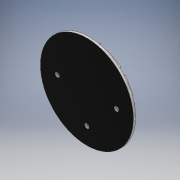
# Autodesk Inventor part: TSSP Receiver
Saved by Autodesk Inventor 2018 (Build 220112000, 112)
## iProperties
Created: 2018-09-04
Part Number: TSSP Receiver
Material: Generic
Document SubType Name: Modeling
Designer: matth
Density: 1 g/cm^3
Appearance: Default
Author: matth
Autodesk Inventor part; units mm, degrees
ref_plane "YZ Plane" through (0, 0, 0) normal (1, 0, 0) x (0, 1, 0)
ref_plane "XZ Plane" through (0, 0, 0) normal (0, 1, 0) x (-1, 0, 0)
ref_plane "XY Plane" through (0, 0, 0) normal (0, 0, 1) x (1, 0, 0)
sketch "Sketch1" plane through (0, 0, 0) normal (0, 1, 0) x (-1, 0, 0)
  line L0 (0, 0) -> (19.05, 0)
  line L1 (0, 0) -> (-19.05, 0)
  line L2 (0, 0) -> (0, -19.05)
  circle A0 centre (-19.05, 0) radius 1.5
  circle A1 centre (19.05, 0) radius 1.5
  circle A2 centre (0, -19.05) radius 1.5
  line L3 (0, -20.55) -> (0, -22.55)
  line L4 (0, -22.55) -> (5, -22.55)
  line L5 (5, -22.55) -> (5, -27.55)
  line L6 (5, -27.55) -> (-5, -27.55)
  line L7 (-5, -27.55) -> (-5, -22.55)
  line L8 (-5, -22.55) -> (0, -22.55)
  circle A3 centre (0, 0) radius 30
  dimension "d6" = 3
  dimension "d0" = 19.05
  dimension "d1" = 19.05
  dimension "d2" = 19.05
  dimension "d4" = 3
  dimension "d5" = 3
  dimension "d7" = 2
  dimension "d8" = 5
  dimension "d9" = 5
  dimension "d10" = 10
  dimension "d11" = 60
  constraints: 18 end point, 4 coincident, 3 centre point, 3 horizontal, 3 perpendicular, 2 vertical, 1 collinear, 1 point on line, 1 vertical alignment, 2 other
  measures "d0" distance of L0.start L0.end
  measures "d1" distance of L0.start L1.end
  measures "d2" distance of L0.start L2.end
  measures "d4" diameter of A0
  measures "d5" diameter of A1
  measures "d7" distance of L3.start L3.end
  measures "d8" distance of L3.end L4.end
  measures "d9" distance of L4.end L5.end
  measures "d10" distance of L5.end L6.end
  measures "d11" diameter of A3
extrude "Extrusion1" add sketch "Sketch1" along normal blind 1.5 contours L4 L5 L6 L7 L8 | A3
sketch "Sketch2" plane through (0, 1.5, 0) normal (0, 1, 0) x (1, 0, 0)
  line L0 (0, 0) -> (0, 22)
  line L1 (0, 22) -> (-5, 22)
  line L2 (-5, 22) -> (-5, 27)
  line L3 (-5, 27) -> (0, 27)
  line L4 (0, 27) -> (5, 27)
  line L5 (5, 27) -> (5, 22)
  line L6 (5, 22) -> (0, 22)
  line L7 (-11, 19.0526) -> (-15.3301, 16.5526)
  line L8 (-15.3301, 16.5526) -> (-17.8301, 20.8827)
  line L9 (-17.8301, 20.8827) -> (-13.5, 23.3827)
  line L10 (-13.5, 23.3827) -> (-9.1699, 25.8827)
  line L11 (-9.1699, 25.8827) -> (-6.6699, 21.5526)
  line L12 (-6.6699, 21.5526) -> (-11, 19.0526)
  line L13 (-19.0526, 11) -> (-21.5526, 6.6699)
  line L14 (-21.5526, 6.6699) -> (-25.8827, 9.1699)
  line L15 (-25.8827, 9.1699) -> (-23.3827, 13.5)
  line L16 (-23.3827, 13.5) -> (-20.8827, 17.8301)
  line L17 (-20.8827, 17.8301) -> (-16.5526, 15.3301)
  line L18 (-16.5526, 15.3301) -> (-19.0526, 11)
  line L19 (-22, 0) -> (-22, -5)
  line L20 (-22, -5) -> (-27, -5)
  line L21 (-27, -5) -> (-27, 0)
  line L22 (-27, 0) -> (-27, 5)
  line L23 (-27, 5) -> (-22, 5)
  line L24 (-22, 5) -> (-22, 0)
  line L25 (-19.0526, -11) -> (-16.5526, -15.3301)
  line L26 (-16.5526, -15.3301) -> (-20.8827, -17.8301)
  line L27 (-20.8827, -17.8301) -> (-23.3827, -13.5)
  line L28 (-23.3827, -13.5) -> (-25.8827, -9.1699)
  line L29 (-25.8827, -9.1699) -> (-21.5526, -6.6699)
  line L30 (-21.5526, -6.6699) -> (-19.0526, -11)
  line L31 (-11, -19.0526) -> (-6.6699, -21.5526)
  line L32 (-6.6699, -21.5526) -> (-9.1699, -25.8827)
  line L33 (-9.1699, -25.8827) -> (-13.5, -23.3827)
  line L34 (-13.5, -23.3827) -> (-17.8301, -20.8827)
  line L35 (-17.8301, -20.8827) -> (-15.3301, -16.5526)
  line L36 (-15.3301, -16.5526) -> (-11, -19.0526)
  line L37 (0, -22) -> (5, -22)
  line L38 (5, -22) -> (5, -27)
  line L39 (5, -27) -> (0, -27)
  line L40 (0, -27) -> (-5, -27)
  line L41 (-5, -27) -> (-5, -22)
  line L42 (-5, -22) -> (0, -22)
  line L43 (11, -19.0526) -> (15.3301, -16.5526)
  line L44 (15.3301, -16.5526) -> (17.8301, -20.8827)
  line L45 (17.8301, -20.8827) -> (13.5, -23.3827)
  line L46 (13.5, -23.3827) -> (9.1699, -25.8827)
  line L47 (9.1699, -25.8827) -> (6.6699, -21.5526)
  line L48 (6.6699, -21.5526) -> (11, -19.0526)
  line L49 (19.0526, -11) -> (21.5526, -6.6699)
  line L50 (21.5526, -6.6699) -> (25.8827, -9.1699)
  line L51 (25.8827, -9.1699) -> (23.3827, -13.5)
  line L52 (23.3827, -13.5) -> (20.8827, -17.8301)
  line L53 (20.8827, -17.8301) -> (16.5526, -15.3301)
  line L54 (16.5526, -15.3301) -> (19.0526, -11)
  line L55 (22, 0) -> (22, 5)
  line L56 (22, 5) -> (27, 5)
  line L57 (27, 5) -> (27, 0)
  line L58 (27, 0) -> (27, -5)
  line L59 (27, -5) -> (22, -5)
  line L60 (22, -5) -> (22, 0)
  line L61 (19.0526, 11) -> (16.5526, 15.3301)
  line L62 (16.5526, 15.3301) -> (20.8827, 17.8301)
  line L63 (20.8827, 17.8301) -> (23.3827, 13.5)
  line L64 (23.3827, 13.5) -> (25.8827, 9.1699)
  line L65 (25.8827, 9.1699) -> (21.5526, 6.6699)
  line L66 (21.5526, 6.6699) -> (19.0526, 11)
  line L67 (11, 19.0526) -> (6.6699, 21.5526)
  line L68 (6.6699, 21.5526) -> (9.1699, 25.8827)
  line L69 (9.1699, 25.8827) -> (13.5, 23.3827)
  line L70 (13.5, 23.3827) -> (17.8301, 20.8827)
  line L71 (17.8301, 20.8827) -> (15.3301, 16.5526)
  line L72 (15.3301, 16.5526) -> (11, 19.0526)
  dimension "d14" = 22
  dimension "d15" = 5
  dimension "d16" = 5
  dimension "d17" = 5
  dimension "d18" = 5
  dimension "d21" = 360
  constraints: 146 end point, 25 point on line, 3 perpendicular, 1 collinear, 1 vertical, 145 other
  measures "d14" distance of L0.start L0.end
  measures "d15" distance of L0.end L1.end
  measures "d16" distance of L1.end L2.end
  measures "d17" distance of L2.end L3.end
  measures "d18" distance of L3.end L4.end
extrude "Extrusion2" add sketch "Sketch2" along normal blind 2.5
body "Solid1"
